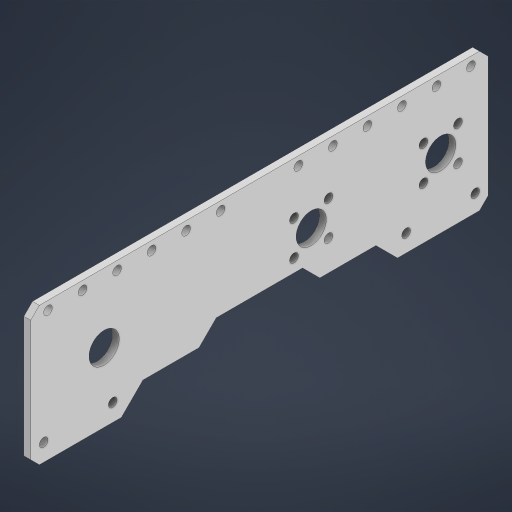
# Autodesk Inventor part: ArmSidePlate_Template
Saved by Autodesk Inventor 2024 (Build 280153000, 153)
## iProperties
Created: 2023-10-25
Part Number: ArmSidePlate_Template
Material: Generic
Document SubType Name: Modeling
Designer: avsar
Density: 1 g/cm^3
Appearance: Default
Author: avsar
Autodesk Inventor part; units mm, degrees
ref_plane "YZ Plane" through (0, 0, 0) normal (1, 0, 0) x (0, 1, 0)
ref_plane "XZ Plane" through (0, 0, 0) normal (0, 1, 0) x (-1, 0, 0)
ref_plane "XY Plane" through (0, 0, 0) normal (0, 0, 1) x (1, 0, 0)
sketch "Sketch1" plane through (0, 0, 0) normal (1, 0, 0) x (0, 1, 0)
  line L0 (-32, 106) -> (32, 106)
  line L1 (32, 106) -> (32, -106)
  line L2 (32, -106) -> (-32, -106)
  line L3 (-32, -106) -> (-32, 106)
  line L4 (-32, 106) -> (32, -106) construction
  line L5 (32, 106) -> (-32, -106) construction
  point P0 (0, 0)
  dimension "d0" = 64
  dimension "d1" = 212
  constraints: 12 end point, 2 midpoint, 2 parallel, 1 horizontal, 1 perpendicular
  measures "d0" distance of L1.end L2.end
  measures "d1" distance of L0.end L1.end
extrude "Extrusion1" add sketch "Sketch1" along normal blind 3.175
chamfer "Chamfer1" distance 4 angle 45 2 edges at (1.5875, 32, 106) (1.5875, 32, -106)
chamfer "Chamfer2" distance 4 angle 45 2 edges at (1.5875, -32, 106) (1.5875, -32, -106)
sketch "Sketch3" plane through (3.175, 0, 0) normal (1, 0, 0) x (0, 0, -1)
  circle A0 centre (-84, -8) radius 7 construction
  circle A1 centre (-68, -24) radius 2
  line L0 (-102, -32) -> (102, -32) construction
  line L1 (-84, -1) -> (-84, -15) construction
  circle A2 centre (-100, -24) radius 2
  line L2 (102, 32) -> (-102, 32) construction
  line L3 (0, 32) -> (0, -32) construction
  circle A3 centre (68, -24) radius 2
  circle A4 centre (100, -24) radius 2
  point P0 (0, 0)
  dimension "d22" = 14
  dimension "d23" = 84
  dimension "d24" = 4
  dimension "d25" = 16
  dimension "d26" = 8
  dimension "d27" = 16
  constraints: 5 centre point, 4 end point, 3 midpoint, 3 symmetric about line, 2 point on circle, 1 coincident, 1 vertical, 3 other
  measures "d22" diameter of A0
  measures "d23" horizontal distance of point (0, 0) A0.centre
  measures "d24" diameter of A1
  measures "d25" horizontal distance of A1.centre A0.centre
  measures "d26" distance from line of L0 A1.centre
  measures "d27" horizontal distance of A1.centre A0.centre
extrude "Extrusion3" cut sketch "Sketch3" against normal through all
sketch "Sketch4" plane through (3.175, 0, 0) normal (1, 0, 0) x (0, 0, -1)
  circle A0 centre (-72, 0) radius 7
  point P0 (0, 0)
  dimension "d30" = 14
  dimension "d31" = 72
  constraints: 1 centre point, 1 horizontal alignment
  measures "d30" diameter of A0
  measures "d31" distance of point (0, 0) A0.centre
extrude "Extrusion4" cut sketch "Sketch4" against normal through all
sketch "Sketch6" plane through (3.175, 0, 0) normal (1, 0, 0) x (0, 0, -1)
  circle A0 centre (-72, 0) radius 7 construction
  circle A1 centre (84, 0) radius 7
  line L0 (84, 0) -> (91, 0) construction
  circle A2 centre (76, 8) radius 2
  circle A3 centre (76, -8) radius 2
  circle A4 centre (92, -8) radius 2
  circle A5 centre (92, 8) radius 2
  circle A6 centre (24, 0) radius 7
  circle A7 centre (16, 8) radius 2
  circle A8 centre (16, -8) radius 2
  circle A9 centre (32, -8) radius 2
  circle A10 centre (32, 8) radius 2
  point P0 (0, 0)
  dimension "d65" = 14
  dimension "d67" = 84
  dimension "d71" = 4
  dimension "d72" = 8
  dimension "d73" = 8
  dimension "d76" = 360
  dimension "d78" = 14
  dimension "d79" = 24
  dimension "d80" = 4
  dimension "d81" = 8
  dimension "d82" = 8
  dimension "d85" = 360
  constraints: 9 centre point, 3 horizontal alignment, 2 end point, 1 horizontal, 20 other
  measures "d67" distance of L0.start point (0, 0)
  measures "d71" diameter of A2
  measures "d72" horizontal distance of L0.start A2.centre
  measures "d73" horizontal distance of L0.start A2.centre
  measures "d78" diameter of A6
  measures "d79" distance of A6.centre point (0, 0)
  measures "d80" diameter of A7
  measures "d81" horizontal distance of A6.centre A7.centre
  measures "d82" horizontal distance of A6.centre A7.centre
extrude "Extrusion6" cut sketch "Sketch6" against normal blind 10
sketch "Sketch8" plane through (3.175, 0, 0) normal (1, 0, 0) x (0, 0, -1)
  circle A0 centre (-98, 28) radius 2
  line L0 (102, 32) -> (-102, 32) construction
  line L1 (-106, 28) -> (-106, -28) construction
  circle A1 centre (-82, 28) radius 2
  circle A2 centre (-66, 28) radius 2
  circle A3 centre (-50, 28) radius 2
  circle A4 centre (-34, 28) radius 2
  circle A5 centre (-18, 28) radius 2
  line L2 (0, 32) -> (0, -32) construction
  line L3 (-102, -32) -> (102, -32) construction
  circle A6 centre (98, 28) radius 2
  circle A7 centre (82, 28) radius 2
  circle A8 centre (66, 28) radius 2
  circle A9 centre (50, 28) radius 2
  circle A10 centre (34, 28) radius 2
  circle A11 centre (18, 28) radius 2
  point P0 (0, 0)
  dimension "d87" = 4
  dimension "d88" = 4
  dimension "d89" = 8
  dimension "d92" = 16
  constraints: 12 centre point, 6 symmetric about line, 2 end point, 2 midpoint, 1 horizontal, 16 other
  measures "d87" diameter of A0
  measures "d88" distance from line of L0 A0.centre
  measures "d89" distance from line of L1 A0.centre
  measures "d92" distance of A0.centre A1.centre
extrude "Extrusion7" cut sketch "Sketch8" against normal through all
sketch "Sketch9" plane through (3.175, 0, 0) normal (1, 0, 0) x (0, 0, -1)
  line L0 (-102, -32) -> (102, -32) construction
  line L1 (-64, -32) -> (-64, -32)
  line L2 (-54, -22) -> (54, -22)
  line L3 (64, -32) -> (64, -32)
  line L4 (-64, -32) -> (64, -32)
  line L5 (-54, -22) -> (-64, -32)
  line L6 (54, -22) -> (64, -32)
  point P0 (0, 0)
  point P1 (-64, -22)
  point P2 (64, -22)
  dimension "d99" = 64
  dimension "d100" = 64
  dimension "d101" = 10
  dimension "d102" = 10
  dimension "d103" = 10
  dimension "d104" = 10
  dimension "d105" = 10
  constraints: 12 end point, 6 point on line, 2 perpendicular, 1 horizontal, 1 vertical
  measures "d99" distance from line of point (0, 0) L1
  measures "d100" distance from line of L3 point (0, 0)
  measures "d101" distance of L1.start point (-64, -22)
  measures "d102" distance of L2.start point (-64, -22)
  measures "d103" distance of L1.end point (-64, -22)
  measures "d104" distance of L2.end point (64, -22)
  measures "d105" distance of L3.start point (64, -22)
extrude "Extrusion8" cut sketch "Sketch9" against normal through all
sketch "Sketch10" plane through (3.175, 0, 0) normal (1, 0, 0) x (0, 0, -1)
  line L0 (-54, -22) -> (54, -22) construction
  line L1 (-28, -22) -> (-28, -22)
  line L2 (-20, -14) -> (20, -14)
  line L3 (28, -22) -> (28, -22)
  line L4 (-28, -22) -> (28, -22)
  line L5 (-20, -14) -> (-28, -22)
  line L6 (20, -14) -> (28, -22)
  point P0 (0, 0)
  point P1 (-28, -14)
  point P2 (28, -14)
  point P3 (0, -14)
  point P4 (0, -22)
  point P5 (28, -22)
  dimension "d108" = 8
  dimension "d109" = 56
  dimension "d110" = 8
  dimension "d111" = 8
  dimension "d112" = 8
  dimension "d113" = 8
  constraints: 12 end point, 5 point on line, 2 midpoint, 2 perpendicular, 1 collinear, 1 vertical, 1 vertical alignment
  measures "d108" distance of L1.start point (-28, -14)
  measures "d109" distance of point (-28, -14) point (28, -14)
  measures "d110" distance of L2.start point (-28, -14)
  measures "d111" distance of L1.end point (-28, -14)
  measures "d112" distance of L2.end point (28, -14)
  measures "d113" distance of L3.start point (28, -14)
extrude "Extrusion9" cut sketch "Sketch10" against normal through all
equation "\"d100\" = d99"
equation "\"d102\" = d101"
equation "\"d103\" = d102"
equation "\"d104\" = d101"
equation "\"d105\" = d104"
equation "\"d110\" = d108"
equation "\"d111\" = d108"
equation "\"d112\" = d108"
equation "\"d113\" = d112"
body "Solid1"
